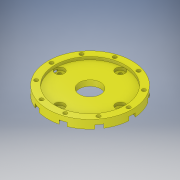
# Autodesk Inventor part: МД.001.201 - Основа
Saved by Autodesk Inventor 2019 (Build 230136000, 136)
## iProperties
Created: 2019-12-22
Part Number: МД.001.201 - Основа
Material: Пластик АБС
Document SubType Name: Modeling
Designer: Петров Иван
Density: 1.06 g/cm^3
Appearance: Желтый
Author: Петров Иван
Autodesk Inventor part; units mm, degrees
ref_plane "YZ Plane" through (0, 0, 0) normal (1, 0, 0) x (0, 1, 0)
ref_plane "XZ Plane" through (0, 0, 0) normal (0, 1, 0) x (-1, 0, 0)
ref_plane "XY Plane" through (0, 0, 0) normal (0, 0, 1) x (1, 0, 0)
sketch "Эскиз1" plane through (0, 0, 0) normal (0, 1, 0) x (-1, 0, 0)
  circle A0 centre (0, 0) radius 45
  circle A1 centre (0, 0) radius 37.5
  dimension "d0" = 90
  dimension "d1" = 75
  constraints: 2 centre point, 2 coincident
  measures "d0" diameter of A0
  measures "d1" diameter of A1
extrude "Выдавливание1" add sketch "Эскиз1" along normal blind 3
sketch "Эскиз2" plane through (0, 0, 0) normal (0, -1, 0) x (1, 0, 0)
  circle A0 centre (0, 0) radius 45
  circle A1 centre (0, 0) radius 45 projected
  circle A2 centre (0, 0) radius 40
  dimension "d4" = 80
  dimension "d5" = 90
  constraints: 2 centre point, 2 coincident
  measures "d4" diameter of A2
  measures "d5" diameter of A0
extrude "Выдавливание2" add sketch "Эскиз2" along normal blind 6 contours A0 | A2
sketch "Эскиз3" plane through (0, 3, 0) normal (0, 1, 0) x (1, 0, 0)
  circle A0 centre (0, 0) radius 37.5 projected
  circle A1 centre (0, 0) radius 45 projected
  circle A2 centre (41.245, 0) radius 2
  line L0 (37.5, 0) -> (37.9725, 0)
  dimension "d10" = 4
  dimension "d30" = 3.745
  constraints: 2 end point, 1 centre point, 1 horizontal, 1 horizontal alignment, 1 other
  measures "d10" diameter of A2
  measures "d30" distance of A2.centre L0.start
extrude "Выдавливание3" cut sketch "Эскиз3" against normal through all contours A2
pattern_circular "Круговой массив1" count 10 over 360 about axis through (0, 0, 0) along (0, 1, 0) of "Выдавливание3"
sketch "Эскиз4" plane through (0, -6, 0) normal (0, -1, 0) x (1, 0, 0)
  circle A0 centre (-33.3679, -24.2432) radius 2 projected
  circle A1 centre (-33.3679, -24.2432) radius 5
  point P0 (0, 0)
  dimension "d16" = 10
  constraints: 1 centre point, 1 coincident
  measures "d16" diameter of A1
extrude "Выдавливание4" cut sketch "Эскиз4" against normal blind 4
pattern_circular "Круговой массив2" count 10 over 360 about axis through (0, 0, 0) along (0, 1, 0) of "Выдавливание4"
sketch "Эскиз5" plane through (0, 0, 0) normal (0, 1, 0) x (1, 0, 0)
  line L0 (15, -27.5) -> (5, -37.5)
  line L1 (5, -37.5) -> (-5, -37.5)
  line L2 (-5, -37.5) -> (-15, -27.5)
  line L3 (-15, -27.5) -> (-27.5, -27.5)
  line L4 (-27.5, -27.5) -> (-27.5, -15)
  line L5 (-27.5, -15) -> (-37.5, -5)
  line L6 (-37.5, -5) -> (-37.5, 5)
  line L7 (-37.5, 5) -> (-27.5, 15)
  line L8 (-27.5, 15) -> (-27.5, 27.5)
  line L9 (-27.5, 27.5) -> (-15, 27.5)
  line L10 (-15, 27.5) -> (-5, 37.5)
  line L11 (-5, 37.5) -> (5, 37.5)
  line L12 (5, 37.5) -> (15, 27.5)
  line L13 (15, 27.5) -> (27.5, 27.5)
  line L14 (27.5, 27.5) -> (27.5, 15)
  line L15 (27.5, 15) -> (37.5, 5)
  line L16 (37.5, 5) -> (37.5, -5)
  line L17 (37.5, -5) -> (27.5, -15)
  line L18 (27.5, -15) -> (27.5, -27.5)
  line L19 (27.5, -27.5) -> (15, -27.5)
  circle A0 centre (0, -32.5) radius 1.9
  circle A1 centre (-32.5, 0) radius 1.9
  circle A2 centre (0, 32.5) radius 1.9
  circle A3 centre (32.5, 0) radius 1.9
  arc A4 (20.5, 15.5) -> (15.5, 20.5) centre (15.5, 15.5) ccw
  arc A5 (15.5, 20.5) -> (10.5, 15.5) centre (15.5, 15.5) ccw
  arc A6 (10.5, 15.5) -> (15.5, 10.5) centre (15.5, 15.5) ccw
  arc A7 (15.5, 10.5) -> (20.5, 15.5) centre (15.5, 15.5) ccw
  arc A8 (-10.5, -15.5) -> (-15.5, -10.5) centre (-15.5, -15.5) ccw
  arc A9 (-15.5, -10.5) -> (-20.5, -15.5) centre (-15.5, -15.5) ccw
  arc A10 (-20.5, -15.5) -> (-15.5, -20.5) centre (-15.5, -15.5) ccw
  arc A11 (-15.5, -20.5) -> (-10.5, -15.5) centre (-15.5, -15.5) ccw
  arc A12 (-10.5, 15.5) -> (-15.5, 20.5) centre (-15.5, 15.5) ccw
  arc A13 (-15.5, 20.5) -> (-20.5, 15.5) centre (-15.5, 15.5) ccw
  arc A14 (-20.5, 15.5) -> (-15.5, 10.5) centre (-15.5, 15.5) ccw
  arc A15 (-15.5, 10.5) -> (-10.5, 15.5) centre (-15.5, 15.5) ccw
  arc A16 (20.5, -15.5) -> (15.5, -10.5) centre (15.5, -15.5) ccw
  arc A17 (15.5, -10.5) -> (10.5, -15.5) centre (15.5, -15.5) ccw
  arc A18 (10.5, -15.5) -> (15.5, -20.5) centre (15.5, -15.5) ccw
  arc A19 (15.5, -20.5) -> (20.5, -15.5) centre (15.5, -15.5) ccw
  arc A20 (11.3, 0) -> (0, 11.3) centre (0, 0) ccw
  arc A21 (0, 11.3) -> (-11.3, 0) centre (0, 0) ccw
  arc A22 (-11.3, 0) -> (0, -11.3) centre (0, 0) ccw
  arc A23 (0, -11.3) -> (11.3, 0) centre (0, 0) ccw
  constraints: 40 end point, 40 point on circle, 24 centre point
extrude "Выдавливание5" cut sketch "Эскиз5" against normal through all contours A0 | A1 | A2 | A3 | A23 A22 A21 A20
sketch "Эскиз6" plane through (0, 0, 0) normal (0, 1, 0) x (1, 0, 0)
  circle A0 centre (32.5, 0) radius 1.9 projected
  circle A1 centre (32.5, 0) radius 5
  point P0 (0, 0)
  dimension "d24" = 10
  constraints: 1 centre point, 1 coincident
  measures "d24" diameter of A1
extrude "Выдавливание6" cut sketch "Эскиз6" against normal blind 3
pattern_circular "Круговой массив3" count 4 over 360 about axis through (0, 0, 0) along (0, -1, 0) of "Выдавливание6"
